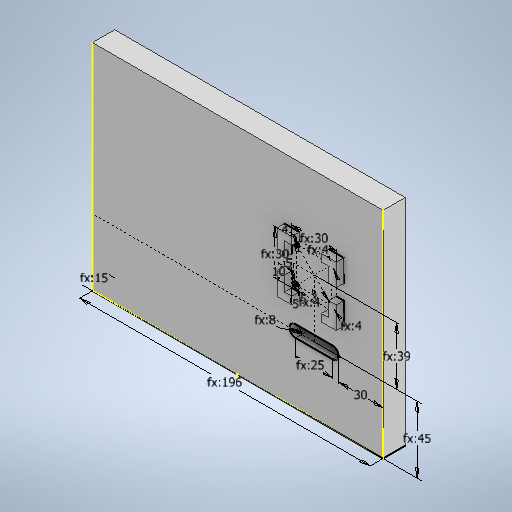
# Autodesk Inventor part: Tapa_frontal
Saved by Autodesk Inventor 2025.1 (Build 291241000, 241)
## iProperties
Created: 2025-11-25
Part Number: Tapa_frontal
Material: Genérico
Document SubType Name: Modeling
Designer: Diego
Density: 1 g/cm^3
Appearance: Valor por defecto
Author: Diego
Autodesk Inventor part; units mm, degrees
ref_plane "YZ Plane" through (0, 0, 0) normal (1, 0, 0) x (0, 1, 0)
ref_plane "XZ Plane" through (0, 0, 0) normal (0, 1, 0) x (-1, 0, 0)
ref_plane "XY Plane" through (0, 0, 0) normal (0, 0, 1) x (1, 0, 0)
sketch "Boceto1" plane through (0, 0, 0) normal (0, 1, 0) x (-1, 0, 0)
  line L0 (-98, -7.5) -> (98, -7.5)
  line L1 (98, -7.5) -> (98, 7.5)
  line L2 (98, 7.5) -> (-98, 7.5)
  line L3 (-98, 7.5) -> (-98, -7.5)
  line L4 (-98, -7.5) -> (98, 7.5) construction
  line L5 (98, -7.5) -> (-98, 7.5) construction
  point P0 (0, 0)
  dimension "d0" = 196
  dimension "d1" = 15
  constraints: 12 end point, 2 midpoint, 2 parallel, 1 horizontal, 1 perpendicular
  measures "d0" distance of L2.end L1.end
  measures "d1" distance of L1.end L0.end
extrude "Extrusión1" add sketch "Boceto1" along normal blind 145
sketch "Boceto3" plane through (0, 0, 0) normal (0, -1, 0) x (1, 0, 0)
  line L0 (-98, -7.5) -> (-98, 7.5) projected
  line L1 (-98, -7.5) -> (-98, 7.5) projected
  line L2 (-98, 7.5) -> (98, 7.5) projected
  line L3 (-98, 7.5) -> (98, 7.5) projected
  line L4 (98, 7.5) -> (98, -7.5) projected
  line L5 (98, 7.5) -> (98, -7.5) projected
  line L6 (98, -7.5) -> (-98, -7.5) projected
  line L7 (98, -7.5) -> (-98, -7.5) projected
  line L8 (-98, -7.5) -> (-98, 7.5) projected
  line L9 (98, -7.5) -> (-98, -7.5) projected
  line L10 (98, 7.5) -> (98, -7.5) projected
  line L11 (-98, 7.5) -> (98, 7.5) projected
  line L12 (-98, -7.5) -> (-98, 7.5) projected
  line L13 (-98, 7.5) -> (98, 7.5) projected
  line L14 (98, 7.5) -> (98, -7.5) projected
  line L15 (98, -7.5) -> (-98, -7.5) projected
  line L16 (-98, -7.5) -> (-98, 7.5) projected
  line L17 (-98, -7.5) -> (-98, 7.5) projected
  line L18 (-98, 7.5) -> (98, 7.5) projected
  line L19 (-98, 7.5) -> (98, 7.5) projected
  line L20 (98, 7.5) -> (98, -7.5) projected
  line L21 (98, 7.5) -> (98, -7.5) projected
  line L22 (98, -7.5) -> (-98, -7.5) projected
  line L23 (98, -7.5) -> (-98, -7.5) projected
  line L24 (98, -7.5) -> (-98, -7.5) projected
  line L25 (-98, -7.5) -> (-98, 7.5) projected
  line L26 (-98, 7.5) -> (98, 7.5) projected
  line L27 (98, 7.5) -> (98, -7.5) projected
  line L28 (98, -7.5) -> (-98, 7.5) construction
  line L29 (-98, -7.5) -> (98, 7.5) construction
  line L30 (90.5, 7.5) -> (90.5, -7.5) construction
  line L31 (88, -7.5) -> (93, -7.5)
  line L32 (88, -7.5) -> (85.5, -3.1699)
  line L33 (85.5, -3.1699) -> (95.5, -3.1699)
  line L34 (95.5, -3.1699) -> (93, -7.5)
  line L35 (0, 7.5) -> (0, -7.5) construction
  line L36 (-88, -7.5) -> (-85.5, -3.1699)
  line L37 (-85.5, -3.1699) -> (-95.5, -3.1699)
  line L38 (-95.5, -3.1699) -> (-93, -7.5)
  point P0 (0, 0)
  point P1 (0, 0)
  point P2 (98, 0)
  dimension "d8" = 7.5
  dimension "d9" = 5
  dimension "d10" = 10
  dimension "d12" = 60
  constraints: 18 end point, 4 symmetric about line, 2 horizontal, 2 midpoint, 1 perpendicular, 11 other
  measures "d8" distance from line of point (98, 0) L30
  measures "d9" distance of L31.start L31.end
  measures "d10" distance of L32.end L33.end
  measures "d12" angle of L32 L33
extrude "Extrusión2" cut sketch "Boceto3" against normal blind 135 contours L38 L37 L36 L6 | L32 L33 L34 L6
sketch "Boceto4" plane through (-98, 0, 7.5) normal (0, 0, 1) x (1, 0, 0)
  line L0 (0, 0) -> (0, 145) projected
  line L1 (0, 45) -> (196, 45) construction
  line L2 (196, 0) -> (196, 145) projected
  line L3 (0, 0) -> (196, 0) projected
  line L4 (162, 45) -> (137, 45) construction
  line L5 (162, 49) -> (137, 49)
  line L6 (137, 41) -> (162, 41)
  arc A0 (162, 41) -> (162, 49) centre (162, 45) ccw
  arc A1 (137, 49) -> (137, 41) centre (137, 45) ccw
  line L7 (149.5, 45) -> (149.5, 84) construction
  line L8 (164.5, 69) -> (134.5, 69) construction
  line L9 (134.5, 69) -> (134.5, 99) construction
  line L10 (134.5, 99) -> (164.5, 99) construction
  line L11 (164.5, 99) -> (164.5, 69) construction
  line L12 (164.5, 69) -> (134.5, 99) construction
  line L13 (134.5, 69) -> (164.5, 99) construction
  line L14 (137.5, 72) -> (161.5, 72) construction
  line L15 (161.5, 72) -> (161.5, 96) construction
  line L16 (161.5, 96) -> (137.5, 96) construction
  line L17 (137.5, 96) -> (137.5, 72) construction
  circle A2 centre (161.5, 96) radius 2
  circle A3 centre (137.5, 96) radius 2
  circle A4 centre (161.5, 72) radius 2
  circle A5 centre (137.5, 72) radius 2
  line L18 (134.5, 69) -> (134.5, 79)
  line L19 (134.5, 79) -> (129.5, 79)
  line L20 (129.5, 79) -> (129.5, 64)
  line L21 (129.5, 64) -> (139.5, 64)
  line L22 (139.5, 64) -> (139.5, 69)
  line L23 (139.5, 69) -> (134.5, 69)
  line L24 (149.5, 84) -> (134.5, 84) construction
  line L25 (134.5, 99) -> (134.5, 89)
  line L26 (134.5, 89) -> (129.5, 89)
  line L27 (129.5, 89) -> (129.5, 104)
  line L28 (129.5, 104) -> (139.5, 104)
  line L29 (139.5, 104) -> (139.5, 99)
  line L30 (139.5, 99) -> (134.5, 99)
  line L31 (164.5, 69) -> (164.5, 79)
  line L32 (164.5, 79) -> (169.5, 79)
  line L33 (169.5, 79) -> (169.5, 64)
  line L34 (169.5, 64) -> (159.5, 64)
  line L35 (159.5, 64) -> (159.5, 69)
  line L36 (159.5, 69) -> (164.5, 69)
  line L37 (164.5, 89) -> (169.5, 89)
  line L38 (169.5, 89) -> (169.5, 104)
  line L39 (164.5, 99) -> (164.5, 89)
  line L40 (169.5, 104) -> (159.5, 104)
  line L41 (159.5, 104) -> (159.5, 99)
  line L42 (159.5, 99) -> (164.5, 99)
  point P0 (98, 0)
  point P1 (166, 45)
  dimension "d15" = 45
  dimension "d16" = 8
  dimension "d17" = 25
  dimension "d18" = 30
  dimension "d22" = 39
  dimension "d23" = 30
  dimension "d24" = 30
  dimension "d25" = 3
  dimension "d27" = 4
  dimension "d28" = 4
  dimension "d29" = 4
  dimension "d30" = 4
  dimension "d31" = 10
  dimension "d32" = 5
  dimension "d33" = 5
  dimension "d34" = 5
  constraints: 82 end point, 15 symmetric about line, 6 centre point, 6 point on line, 5 parallel, 5 point on circle, 4 coincident, 4 horizontal, 4 midpoint, 4 perpendicular, 4 tangent, 1 vertical, 3 other
  measures "d15" distance between parallel lines of L3 L1
  measures "d16" diameter of A1
  measures "d17" distance of L6.start L6.end
  measures "d18" distance from line of L2 point (166, 45)
  measures "d22" distance of L7.start L7.end
  measures "d23" distance of L9.end L10.end
  measures "d24" distance of L8.end L9.end
  measures "d25" distance between parallel lines of L8 L14
  measures "d27" diameter of A2
  measures "d28" diameter of A3
  measures "d29" diameter of A4
  measures "d30" diameter of A5
  measures "d31" distance of L8.end L18.end
  measures "d32" distance of L21.end L22.end
  measures "d33" distance of L22.end L8.end
  measures "d34" distance of L18.end L19.end
extrude "Extrusión3" cut sketch "Boceto4" against normal through all contours A0 L6 A1 L5
fillet "Empalme1" radius 0.1 4 edges at (93, 67.5, -7.5) (88, 67.5, -7.5) (-88, 67.5, -7.5) (-93, 67.5, -7.5)
extrude "Extrusión4" cut sketch "Boceto4" against normal blind 10 contours A2 | A3 | A4 | A5
extrude "Extrusión5" add sketch "Boceto4" along normal blind 5 contours L23 L22 L21 L20 L19 L18 | L25 L26 L27 L28 L29 L30 | L31 L32 L33 L34 L35 L36 | L39 L42 L41 L40 L38 L37
equation "\"d27\" = d28"
equation "\"d29\" = d28"
equation "\"d30\" = d28"
